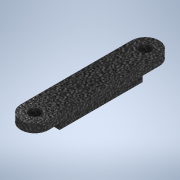
# Autodesk Inventor part: магнит 2
Saved by Autodesk Inventor 2020.1 (Build 241239000, 239)
## iProperties
Created: 2021-10-28
Part Number: магнит 2
Material: Сталь
Document SubType Name: Modeling
Designer: Ni3na
Density: 7.85 g/cm^3
Appearance: Черный — литой
Author: Ni3na
Autodesk Inventor part; units mm, degrees
ref_plane "YZ Plane" through (0, 0, 0) normal (1, 0, 0) x (0, 1, 0)
ref_plane "XZ Plane" through (0, 0, 0) normal (0, 1, 0) x (-1, 0, 0)
ref_plane "XY Plane" through (0, 0, 0) normal (0, 0, 1) x (1, 0, 0)
sketch "Эскиз1" plane through (0, 0, 0) normal (0, 1, 0) x (-1, 0, 0)
  line L0 (-11.1966, 15.641) -> (-1.1966, 15.641)
  line L1 (-1.1966, 15.641) -> (-1.1966, -34.359)
  line L2 (-1.1966, -34.359) -> (-11.1966, -34.359)
  line L3 (-11.1966, -34.359) -> (-11.1966, 15.641)
  point P0 (0, 0)
  dimension "d0" = 50
  dimension "d1" = 10
  constraints: 8 end point, 2 parallel, 1 horizontal, 1 perpendicular
  measures "d0" distance of L2.end L0.start
  measures "d1" distance of L0.start L0.end
extrude "Выдавливание1" add sketch "Эскиз1" along normal blind 3
fillet "Сопряжение1" radius 5 2 edges at (11.1966, 1.5, -34.359) (1.1966, 1.5, -34.359)
fillet "Сопряжение2" radius 5 2 edges at (11.1966, 1.5, 15.641) (1.1966, 1.5, 15.641)
sketch "Эскиз2" plane through (0, 3, 0) normal (0, 1, 0) x (1, 0, 0)
  line L0 (2.1966, 24.359) -> (10.1966, 24.359)
  line L1 (10.1966, 24.359) -> (10.1966, -5.641)
  line L2 (10.1966, -5.641) -> (2.1966, -5.641)
  line L3 (2.1966, -5.641) -> (2.1966, 24.359)
  arc A0 (11.1966, 29.359) -> (1.1966, 29.359) centre (6.1966, 29.359) ccw projected
  arc A1 (1.1966, -10.641) -> (11.1966, -10.641) centre (6.1966, -10.641) ccw projected
  line L4 (11.1966, -10.641) -> (11.1966, 29.359) projected
  line L5 (1.1966, 29.359) -> (1.1966, -10.641) projected
  point P0 (0, 0)
  point P1 (6.1966, 34.359)
  point P2 (6.1966, 24.359)
  point P3 (6.1966, -15.641)
  point P4 (6.1966, -5.641)
  dimension "d6" = 10
  dimension "d7" = 10
  dimension "d8" = 1
  dimension "d9" = 1
  constraints: 8 end point, 2 midpoint, 2 parallel, 2 point on circle, 1 coincident, 1 horizontal, 1 perpendicular
  measures "d6" distance of point (6.197, 24.359) point (6.197, 34.359)
  measures "d7" distance of point (6.197, -5.641) point (6.197, -15.641)
  measures "d8" distance between parallel lines of L4 L1
  measures "d9" distance between parallel lines of L5 L3
extrude "Выдавливание2" cut sketch "Эскиз2" against normal blind 0.1 contours L0 L1 L2 L3
sketch "Эскиз3" plane through (0, 3, 0) normal (0, 1, 0) x (1, 0, 0)
  circle A0 centre (23.3894, 111.2567) radius 1
  circle A1 centre (6.1966, 29.359) radius 2
  arc A2 (11.1966, 29.359) -> (1.1966, 29.359) centre (6.1966, 29.359) ccw projected
  circle A3 centre (6.1966, -10.641) radius 2
  arc A4 (1.1966, -10.641) -> (11.1966, -10.641) centre (6.1966, -10.641) ccw projected
  point P0 (0, 0)
  point P1 (6.1966, 34.359)
  point P2 (6.1966, -15.641)
  dimension "d12" = 2
  dimension "d13" = 4
  dimension "d14" = 5
  dimension "d15" = 4
  constraints: 3 centre point, 2 coincident, 2 point on circle
  measures "d12" diameter of A0
  measures "d13" diameter of A1
  measures "d14" distance of A1.centre point (6.197, 34.359)
  measures "d15" diameter of A3
extrude "Выдавливание3" cut sketch "Эскиз3" against normal blind 10 contours A1 | A3
sketch "Эскиз4" plane through (0, 0, 0) normal (0, -1, 0) x (1, 0, 0)
  line L0 (10.1966, 5.641) -> (2.1966, 5.641) projected
  line L1 (2.1966, 5.641) -> (2.1966, -24.359) projected
  line L2 (10.1966, 5.641) -> (2.1966, 5.641)
  line L3 (2.1966, 5.641) -> (2.1966, -24.359)
  line L4 (2.1966, -24.359) -> (10.1966, -24.359)
  line L5 (10.1966, -24.359) -> (10.1966, 5.641)
  point P0 (0, 0)
  constraints: 8 end point, 2 parallel, 1 horizontal, 1 perpendicular
extrude "Выдавливание4" add sketch "Эскиз4" along normal blind 3
